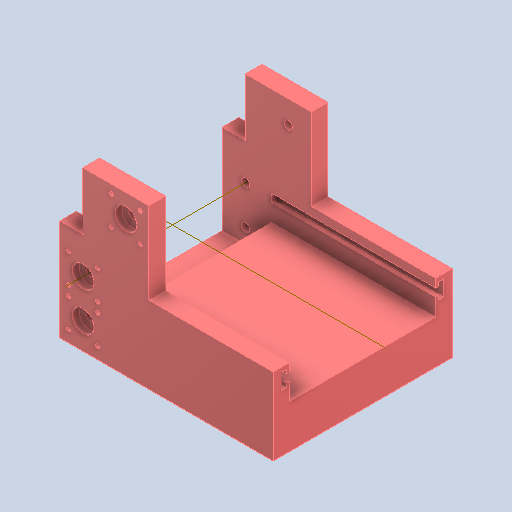
# Autodesk Inventor part: Type 1A R1前充座:1
Saved by Autodesk Inventor 2025 (Build 290162000, 162)
## iProperties
Created: 2024-09-22
Part Number: Type 1A R1前充座:1
Material: 密度7850的鋼
Document SubType Name: Modeling
Designer: veter
Density: 7.84999 g/cm^3
Appearance: 平滑 - 紅色
Mass: 1.98367e+06 g
Surface Area: 50957.3 cm^2
Volume: 252697 cm^3
Stock Number: 1
Author: veter
Autodesk Inventor part; units mm, degrees
ref_plane "YZ Plane" through (0, 0, 0) normal (1, 0, 0) x (0, 1, 0)
ref_plane "XZ Plane" through (0, 0, 0) normal (0, 1, 0) x (-1, 0, 0)
ref_plane "XY Plane" through (0, 0, 0) normal (0, 0, 1) x (1, 0, 0)
sketch "草圖1" plane through (0, 0, 0) normal (0, 0, 1) x (0, 1, 0)
  line L0 (-335, 120) -> (190, 120)
  line L1 (190, 120) -> (190, -135)
  line L2 (190, -135) -> (65, -135)
  line L3 (65, -135) -> (65, -985.5331)
  line L4 (65, -985.5331) -> (-335, -985.5331)
  line L5 (-335, -985.5331) -> (-335, 120)
  line L6 (0, 0) -> (0, -585.5331) construction
  dimension "d0" = 120
  dimension "d2" = 335
  dimension "d3" = 255
  dimension "d4" = 525
  dimension "d13" = 585.5331
  dimension "d14" = 400
  dimension "d15" = 400
  constraints: 14 end point, 5 perpendicular, 1 horizontal, 1 vertical
  measures "d0" distance from line of L0 L6.start
  measures "d2" distance from line of L6.start L5
  measures "d3" distance of L0.end L1.end
  measures "d4" distance of L0.start L0.end
  measures "d13" distance of L6.start L6.end
  measures "d14" distance of L3.end L4.end
  measures "d15" distance from line of L4 L6.end
extrude "擠出1" add sketch "草圖1" along normal mid plane 928
sketch "草圖2" plane through (135, 190, 464) normal (1, 0, 0) x (0, 0, -1)
  line L0 (842, 1535) -> (86, 1535)
  line L1 (86, 1535) -> (86, -465)
  line L2 (86, -465) -> (842, -465)
  line L3 (842, -465) -> (842, 1535)
  line L4 (0, -525) -> (928, -525) projected
  line L5 (928, -125) -> (928, -525) projected
  point P0 (464, -190)
  point P1 (464, -465)
  dimension "d18" = 60
  dimension "d19" = 86
  dimension "d52" = 2000
  constraints: 8 end point, 2 parallel, 1 horizontal, 1 midpoint, 1 perpendicular, 1 vertical alignment
  measures "d18" distance between parallel lines of L4 L2
  measures "d19" distance between parallel lines of L5 L3
  measures "d52" distance of L0.end L1.end
extrude "擠出2" cut sketch "草圖2" against normal through all
sketch "草圖3" plane through (135, 190, 464) normal (-1, 0, 0) x (0, 0, 1)
  line L0 (-842, -125) -> (-86, -125) projected
  line L1 (-842, -465) -> (-842, -125) projected
  line L2 (-86, -465) -> (-842, -465) projected
  line L3 (-86, -125) -> (-86, -465) projected
  line L4 (-842, -300) -> (-86, -300)
  line L5 (0, -525) -> (-928, -525) projected
  point P0 (-464, -190)
  dimension "d60" = 225
  constraints: 2 end point, 2 point on line, 1 horizontal
  measures "d60" distance between parallel lines of L5 L4
extrude "擠出3" cut sketch "草圖3" against normal through all contours L0 L3 L4 L1
fillet "圓角1" radius 60 2 edges at (135, 65, 421) (135, 65, -421)
fillet "圓角2" radius 60 1 edges at (135, -275, 0)
sketch "草圖7" plane through (0, 0, 464) normal (0, 0, 1) x (1, 0, 0)
  line L0 (195, 65) -> (985.5331, 65) projected
  line L1 (135, 190) -> (135, 125) projected
  arc A0 (135, 125) -> (195, 65) centre (195, 125) ccw projected
  line L2 (195, 65) -> (985.5331, 65) projected
  line L3 (985.5331, 65) -> (985.5331, -335) projected
  line L4 (985.5331, -335) -> (-120, -335) projected
  line L5 (-120, 190) -> (135, 190) projected
  line L6 (-120, -335) -> (-120, 190) projected
  line L7 (0, 0) -> (341.7475, 0)
  line L8 (341.7475, 0) -> (341.7475, 489.2781)
  line L9 (341.7475, 489.2781) -> (0, 489.2781)
  line L10 (0, 489.2781) -> (0, 0)
  line L11 (-120, 190) -> (-120, -335) projected
  point P0 (341.7475, 65)
  point P1 (0, 190)
  point P2 (164.4032, 73.3876)
  dimension "d61" = -341.7475
  dimension "d62" = 489.2781
  constraints: 8 end point, 2 parallel, 1 horizontal, 1 perpendicular
  measures "d61" distance of L8.end L9.end
  measures "d62" distance of L7.end L8.end
extrude "擠出7" add sketch "草圖7" against normal up to surface (86 mm away) contours A0 L1 L5 L10 L9 L8 L0 | L0 L8 L7 L10 L5 L1 A0
sketch "草圖4" plane through (0, 0, 464) normal (0, 0, 1) x (1, 0, 0)
  line L0 (-75, -75) -> (75, -75) construction
  line L1 (75, -75) -> (75, 75) construction
  line L2 (75, 75) -> (-75, 75) construction
  line L3 (-75, 75) -> (-75, -75) construction
  line L4 (-75, -75) -> (75, 75) construction
  line L5 (75, -75) -> (-75, 75) construction
  circle A0 centre (0, 0) radius 56.25
  circle A1 centre (75, 75) radius 10.2
  circle A2 centre (75, -75) radius 10.2
  circle A3 centre (-75, -75) radius 10.2
  circle A4 centre (-75, 75) radius 10.2
  line L6 (-75, -275) -> (75, -275) construction
  line L7 (75, -275) -> (75, -125) construction
  line L8 (75, -125) -> (-75, -125) construction
  line L9 (-75, -125) -> (-75, -275) construction
  line L10 (-75, -275) -> (75, -125) construction
  line L11 (75, -275) -> (-75, -125) construction
  circle A5 centre (0, -200) radius 56.25
  circle A6 centre (75, -125) radius 10.2
  circle A7 centre (75, -275) radius 10.2
  circle A8 centre (-75, -275) radius 10.2
  circle A9 centre (-75, -125) radius 10.2
  line L12 (146.7475, 294.2781) -> (296.7475, 294.2781) construction
  line L13 (296.7475, 294.2781) -> (296.7475, 444.2781) construction
  line L14 (296.7475, 444.2781) -> (146.7475, 444.2781) construction
  line L15 (146.7475, 444.2781) -> (146.7475, 294.2781) construction
  line L16 (146.7475, 294.2781) -> (296.7475, 444.2781) construction
  line L17 (296.7475, 294.2781) -> (146.7475, 444.2781) construction
  circle A10 centre (221.7475, 369.2781) radius 56.25
  circle A11 centre (296.7475, 444.2781) radius 10.2
  circle A12 centre (296.7475, 294.2781) radius 10.2
  circle A13 centre (146.7475, 294.2781) radius 10.2
  circle A14 centre (146.7475, 444.2781) radius 10.2
  line L18 (-120, -335) -> (985.5331, -335) projected
  point P0 (-270.371, -335)
  dimension "d27" = 150
  dimension "d28" = 112.5
  dimension "d29" = 20.4
  dimension "d30" = 150
  dimension "d31" = 112.5
  dimension "d32" = 20.4
  dimension "d33" = 150
  dimension "d34" = 112.5
  dimension "d35" = 20.4
  dimension "d36" = 704.2781
  dimension "d37" = -221.7475
  dimension "d38" = 200
  constraints: 36 end point, 16 coincident, 15 centre point, 9 equal radius, 6 midpoint, 6 parallel, 6 perpendicular, 3 horizontal, 1 vertical alignment
  measures "d27" distance of L2.end L1.end
  measures "d28" diameter of A0
  measures "d29" diameter of A1
  measures "d30" distance of L8.end L7.end
  measures "d31" diameter of A5
  measures "d32" diameter of A6
  measures "d33" distance of L14.end L13.end
  measures "d34" diameter of A10
  measures "d35" diameter of A11
  measures "d36" distance from line of L18 point (221.748, 369.278)
  measures "d37" horizontal distance of point (0, 0) point (221.748, 369.278)
  measures "d38" distance of point (0, 0) point (0, -200)
extrude "擠出4" cut sketch "草圖4" against normal blind 36
sketch "草圖5" plane through (0, 0, 428) normal (0, 0, 1) x (1, 0, 0)
  circle A0 centre (75, -75) radius 10.2 projected
  circle A1 centre (-75, -75) radius 10.2 projected
  line L0 (985.5331, 65) -> (985.5331, -335) projected
  line L1 (985.5331, -335) -> (-120, -335) projected
  circle A2 centre (0, 0) radius 21.25
  circle A3 centre (75, 75) radius 10.2 projected
  circle A4 centre (0, 0) radius 56.25 projected
  circle A5 centre (75, -125) radius 10.2 projected
  circle A6 centre (-75, 75) radius 10.2 projected
  circle A7 centre (-75, -275) radius 10.2 projected
  circle A8 centre (75, -275) radius 10.2 projected
  circle A9 centre (-75, -125) radius 10.2 projected
  circle A10 centre (0, -200) radius 56.25 projected
  line L2 (341.7475, 65) -> (985.5331, 65) projected
  circle A11 centre (221.7475, 369.2781) radius 21.25
  circle A12 centre (0, -200) radius 21.25
  line L3 (-120, -335) -> (-120, 190) projected
  line L4 (341.7475, 489.2781) -> (341.7475, 65) projected
  line L5 (-120, 190) -> (0, 190) projected
  line L6 (0, 190) -> (0, 489.2781) projected
  line L7 (0, 489.2781) -> (341.7475, 489.2781) projected
  circle A13 centre (146.7475, 294.2781) radius 10.2 projected
  circle A14 centre (221.7475, 369.2781) radius 56.25 projected
  circle A15 centre (296.7475, 444.2781) radius 10.2 projected
  circle A16 centre (296.7475, 294.2781) radius 10.2 projected
  circle A17 centre (146.7475, 444.2781) radius 10.2 projected
  point P0 (-240, 920)
  point P1 (150.371, 550)
  point P2 (370, 250)
  dimension "d42" = 42.5
  dimension "d54" = 42.5
  dimension "d55" = 42.5
  dimension "d63" = -221.7475
  dimension "d64" = 369.2781
  constraints: 3 centre point, 3 coincident
  measures "d42" diameter of A2
  measures "d54" diameter of A11
  measures "d55" diameter of A12
  measures "d63" horizontal distance of point (0, 0) point (221.748, 369.278)
  measures "d64" vertical distance of point (0, 0) point (221.748, 369.278)
extrude "擠出5" cut sketch "草圖5" against normal blind 60 contours A2 | A11 | A12
sketch "草圖6" plane through (985.5331, -335, 464) normal (1, 0, 0) x (0, 0, -1)
  line L0 (86, 355.25) -> (68.5, 355.25)
  line L1 (68.5, 355.25) -> (68.5, 376.25)
  line L2 (68.5, 376.25) -> (42.5, 376.25)
  line L3 (42.5, 376.25) -> (42.5, 293.75)
  line L4 (42.5, 293.75) -> (68.5, 293.75)
  line L5 (68.5, 293.75) -> (68.5, 314.75)
  line L6 (68.5, 314.75) -> (86, 314.75)
  line L7 (86, 225) -> (86, 400) projected
  point P0 (464, 335)
  point P1 (42.5, 335)
  dimension "d46" = 82.5
  dimension "d47" = 26
  dimension "d48" = 40.5
  dimension "d49" = 17.5
  constraints: 14 end point, 5 perpendicular, 4 point on line, 1 collinear, 1 horizontal, 1 horizontal alignment, 1 midpoint
  measures "d46" distance of L2.end L3.end
  measures "d47" distance of L1.end L2.end
  measures "d48" distance between parallel lines of L6 L0
  measures "d49" distance of L0.start L0.end
extrude "擠出6" cut sketch "草圖6" against normal up to surface (850.5331 mm away)
mirror "鏡射2" about plane through (0, 0, 0) normal (0, 0, 1) of "擠出4", "擠出5", "擠出6", "擠出7"
equation "\"d13\" = R1"
equation "\"d36\" = d2 + R8"
equation "\"R1\" = 585.5331"
equation "\"R7\" = -221.7475"
equation "\"R8\" = 369.2781"
equation "\"Width\" = 756"
equation "\"T1A_R1\" = 585.5331"
equation "\"T1A_R7\" = -221.7475"
equation "\"T1A_R8\" = 369.2781"
equation "\"T1A_R1_Width\" = 756"
equation "\"T1A_R3\" = 252.3048"
equation "\"T1A_R4\" = 320.6953"
equation "\"T1A_R5\" = 419.3047"
equation "\"T1A_R2_Width\" = 756"
equation "\"T1A_R3_Width\" = 344"
equation "\"T1A_R4_Width\" = 756"
equation "\"T1A_Joint_Width\" = 756"
